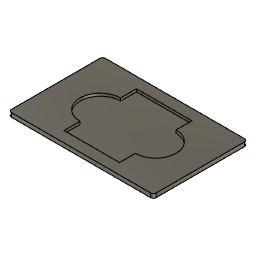
Wingspan - Nectar Lid (Autodesk Fusion 360 design; units mm, degrees)
Autodesk Fusion 360 part; units mm, degrees
note: some values were not read from the file. Set by a fixed rule: which sketch regions a step uses.
sketch "Skizze1" plane through (0, 0, 0) normal (0, 0, 1) x (1, 0, 0)
  line L0 (0, 0) -> (107, 0)
  line L1 (107, 0) -> (107, 69.5)
  line L2 (107, 69.5) -> (0, 69.5)
  line L3 (0, 69.5) -> (0, 0)
  dimension "d1" = 107
  dimension "d2" = 69.5
  constraint horizontal L0
  constraint vertical L1
  constraint horizontal L2
  constraint vertical L3
  constraint coincident L0.start L3.end
  measures "d1" distance of L0.start L0.end
  measures "d2" distance of L0.start L2.end
extrude "Extrusion1" add sketch "Skizze1" along normal blind 3
sketch "Skizze2" plane through (0, 0, 0) normal (0, 0, -1) x (1, 0, 0)
  line L0 (0, 0) -> (0, -69.5)
  line L1 (0, -69.5) -> (107, -69.5)
  line L2 (107, -69.5) -> (107, 0)
  line L3 (107, 0) -> (0, 0)
  line L4 (0, 0) -> (7, 0)
  line L5 (7, 0) -> (7, -7)
  line L6 (7, -7) -> (0, -7)
  line L7 (0, -7) -> (0, 0)
  line L8 (107, 0) -> (100, 0)
  line L9 (100, 0) -> (100, -7)
  line L10 (100, -7) -> (107, -7)
  line L11 (107, -7) -> (107, 0)
  line L12 (107, -69.5) -> (100, -69.5)
  line L13 (100, -69.5) -> (100, -62.5)
  line L14 (100, -62.5) -> (107, -62.5)
  line L15 (107, -62.5) -> (107, -69.5)
  line L16 (0, -69.5) -> (7, -69.5)
  line L17 (7, -69.5) -> (7, -62.5)
  line L18 (7, -62.5) -> (0, -62.5)
  line L19 (0, -62.5) -> (0, -69.5)
  circle A0 centre (3.5, -66) radius 2.65
  circle A1 centre (103.5, -66) radius 2.65
  circle A2 centre (103.5, -3.5) radius 2.65
  circle A3 centre (3.5, -3.5) radius 2.65
  dimension "d5" = 7
  dimension "d6" = 7
  dimension "d7" = 7
  dimension "d8" = 7
  dimension "d9" = 7
  dimension "d10" = 7
  dimension "d11" = 7
  dimension "d12" = 7
  dimension "d13" = 5.3
  dimension "d14" = 5.3
  dimension "d15" = 5.3
  dimension "d16" = 5.3
  dimension "d17" = 3.5
  dimension "d18" = 3.5
  dimension "d19" = 3.5
  dimension "d20" = 3.5
  dimension "d21" = 3.5
  dimension "d22" = 3.5
  dimension "d23" = 3.5
  dimension "d24" = 3.5
  constraint horizontal L4
  constraint vertical L5
  constraint horizontal L6
  constraint vertical L7
  constraint coincident L0.start L3.end
  constraint horizontal L8
  constraint vertical L9
  constraint horizontal L10
  constraint vertical L11
  constraint coincident L2.end L3.start
  constraint horizontal L12
  constraint vertical L13
  constraint horizontal L14
  constraint vertical L15
  constraint coincident L1.end L2.start
  constraint horizontal L16
  constraint vertical L17
  constraint horizontal L18
  constraint vertical L19
  constraint coincident L0.end L1.start
  measures "d5" distance of L0.start L4.end
  measures "d6" distance of L0.start L6.end
  measures "d7" distance of L2.end L8.end
  measures "d8" distance of L2.end L10.end
  measures "d9" distance of L1.end L12.end
  measures "d10" distance of L1.end L14.end
  measures "d11" distance of L0.end L16.end
  measures "d12" distance of L0.end L18.end
  measures "d13" diameter of A0
  measures "d14" diameter of A1
  measures "d15" diameter of A2
  measures "d16" diameter of A3
  measures "d17" distance of L4 A3.centre
  measures "d18" distance of L7 A3.centre
  measures "d19" distance of L11 A2.centre
  measures "d20" distance of L8 A2.centre
  measures "d21" distance of L14 A1.centre
  measures "d22" distance of L15 A1.centre
  measures "d23" distance of L16 A0.centre
  measures "d24" distance of L19 A0.centre
extrude "Extrusion2" cut sketch "Skizze2" against normal blind 1.2 contours A0 | A1 | A2 | A3
fillet "Abrundung1" radius 2 4 edges at (0, 0, 1.5) (107, 0, 1.5) (107, 69.5, 1.5) (0, 69.5, 1.5)
sketch "Skizze3" plane through (0, 0, 3) normal (0, 0, 1) x (-1, 0, 0)
  arc A0 (-2, -69.5) -> (0, -67.5) centre (-2, -67.5) ccw
  line L0 (0, -67.5) -> (0, -2)
  arc A1 (0, -2) -> (-2, 0) centre (-2, -2) ccw
  line L1 (-2, 0) -> (-105, 0)
  arc A2 (-105, 0) -> (-107, -2) centre (-105, -2) ccw
  line L2 (-107, -2) -> (-107, -67.5)
  arc A3 (-107, -67.5) -> (-105, -69.5) centre (-105, -67.5) ccw
  line L3 (-105, -69.5) -> (-2, -69.5)
  line L4 (-33, -61.5) -> (-74, -61.5)
  line L5 (-74, -61.5) -> (-74, -8)
  line L6 (-74, -8) -> (-33, -8)
  line L7 (-33, -8) -> (-33, -61.5)
  circle A4 centre (-33, -34.75) radius 15
  circle A5 centre (-74, -34.75) radius 15
  dimension "d29" = 41
  dimension "d30" = 53.5
  dimension "d31" = 33
  dimension "d32" = 8
  dimension "d33" = 30
  dimension "d34" = 30
  constraint horizontal L4
  constraint vertical L5
  constraint horizontal L6
  constraint vertical L7
  constraint midpoint L7 A4.centre
  constraint midpoint L5 A5.centre
  measures "d29" distance of L4.start L4.end
  measures "d30" distance of L4.start L6.end
  measures "d31" distance of L0 L7
  measures "d32" distance of L1 L6
  measures "d33" diameter of A4
  measures "d34" diameter of A5
extrude "Extrusion3" cut sketch "Skizze3" against normal blind 2 contours L4 L5 L6 L7 A4 A5 | L7 A4 | L7 A4 | L5 A5 | L5 A5
equation "d31 = ( ( 74 / 2 ) * 1 mm ) - 4 mm"
